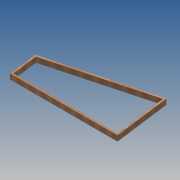
# Autodesk Inventor part: panelBflat
Saved by Autodesk Inventor 2014 SP1 (Build 180222100, 222)
## iProperties
Created: 2015-02-12
Part Number: panelBflat
Material: Wood (Birch)
Document SubType Name: Modeling
Designer: Dave
Density: 0.55 g/cm^3
Appearance: Birch - Natural Polished
Mass: 14992.5 g
Surface Area: 19129.1 cm^2
Volume: 27259 cm^3
Author: Dave
Autodesk Inventor part; units mm, degrees
ref_plane "YZ Plane" through (0, 0, 0) normal (1, 0, 0) x (0, 1, 0)
ref_plane "XZ Plane" through (0, 0, 0) normal (0, 1, 0) x (-1, 0, 0)
ref_plane "XY Plane" through (0, 0, 0) normal (0, 0, 1) x (1, 0, 0)
sketch "Sketch1" plane through (0, 0, 0) normal (0, 1, 0) x (-1, 0, 0)
  line L0 (0, 0) -> (-4153.4811, -1112.9219) construction
  line L1 (0, 0) -> (4300, 0) construction
  line L2 (-4300, 0) -> (-4200, 0) construction
  line L3 (-2006.9086, 50) -> (-4302.025, 50)
  line L4 (-4153.4811, -1112.9219) -> (-3780.7254, -1112.9219) construction
  line L5 (-1925.5839, -567.7225) -> (-4142.0661, -1161.6271)
  line L6 (-4151.9012, -1124.9219) -> (-4302.025, 15.3817)
  line L7 (-1930.5867, -529.7225) -> (-2001.9058, 12)
  line L8 (-4263.2519, 12) -> (-2040.2337, 12)
  line L9 (-2040.2337, 12) -> (-1967.6086, -539.6424)
  line L10 (-1967.6086, -539.6424) -> (-4114.8793, -1115.0019)
  line L11 (-4114.8793, -1115.0019) -> (-4263.2519, 12)
  line L12 (-2006.9086, 50) -> (-2001.9058, 50)
  line L13 (-2040.2337, 12) -> (-1982.3344, 12) construction
  line L14 (-2001.9058, 12) -> (-2001.9058, 50)
  line L15 (-1967.6086, -539.6424) -> (-1881.5519, -516.5836) construction
  line L16 (-1930.5867, -529.7225) -> (-1920.5811, -567.0638)
  line L17 (-1920.5811, -567.0638) -> (-1925.5839, -567.7225)
  line L18 (-4263.2519, 12) -> (-4318.8305, 12) construction
  line L19 (-4302.025, 15.3817) -> (-4302.025, 50)
  line L20 (-4114.8793, -1115.0019) -> (-4170.6932, -1129.9572) construction
  line L21 (-4151.9012, -1124.9219) -> (-4142.0661, -1161.6271)
  dimension "d0" = 4300
  dimension "d1" = 4300
  dimension "d2" = 165
  dimension "d7" = 50
  dimension "d11" = 38
  constraints: 44 end point, 7 perpendicular, 5 point on line, 3 horizontal, 3 parallel, 1 collinear, 1 equal length
  measures "d0" distance of L0.start L2.start
  measures "d1" distance of L0.start L0.end
  measures "d2" angle of L0 L1
  measures "d7" distance between parallel lines of L5 L0
  measures "d11" distance between parallel lines of L8 L3
extrude "Extrusion2" add sketch "Sketch1" along normal blind 114
sketch "Sketch2" plane through (0, 114, 0) normal (0, 1, 0) x (1, 0, 0)
  line L0 (2040.2337, -12) -> (1967.6086, 539.6424) projected
  line L1 (2001.9058, -50) -> (4302.025, -50) projected
  line L2 (4142.0661, 1161.6271) -> (1925.5839, 567.7225) projected
  line L3 (1925.5839, 567.7225) -> (2001.9058, -12) projected
  line L4 (1967.6086, 539.6424) -> (1930.5867, 529.7225)
  line L5 (2040.2337, -12) -> (2001.9058, -12)
  point P0 (2006.9086, -50)
  point P1 (0, 0)
  constraints: 5 end point, 2 parallel, 1 point on line
extrude "Extrusion3" cut sketch "Sketch2" against normal blind 1
sketch "Sketch7" plane through (0, 114, 0) normal (0, 1, 0) x (1, 0, 0)
  line L0 (4114.8793, 1115.0019) -> (4263.2519, -12) projected
  line L1 (4302.025, -50) -> (4302.025, -15.3817) projected
  line L2 (4302.025, -15.3817) -> (4151.9012, 1124.9219) projected
  line L3 (1920.5811, 567.0638) -> (1930.5867, 529.7225) projected
  line L4 (4263.2519, -12) -> (4301.5798, -12)
  line L5 (4114.8793, 1115.0019) -> (4151.9012, 1124.9219)
  point P0 (0, 0)
  constraints: 4 end point, 2 perpendicular, 1 point on line
extrude "Extrusion6" cut sketch "Sketch7" against normal blind 1
body "Solid2"
